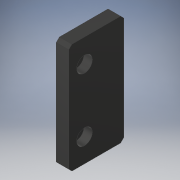
# Autodesk Inventor part: BT503_trajan20_21
Saved by Autodesk Inventor 2022.2 (Build 262287000, 287)
## iProperties
Company: HTBLA Kaindorf
RuleStatus: InUse
Created: 2022-08-19
Part Number: BT503_trajan20_21
Project: Zeichenmaschine_v2
Material: Kunststoff, undurchsichtig Schwarz
Description: Stifthalter_platte
Document SubType Name: Modeling
Designer: trajan20
Density: 0.952 g/cm^3
Appearance: Glatt - Schwarz
Mass: 17.4692 g
Surface Area: 70.5744 cm^2
Volume: 18.35 cm^3
AfterDocNew0: iProperties-Editor_aufrufen
Author: jan
Keywords: 2021
Autodesk Inventor part; units mm, degrees
ref_plane "YZ Plane" through (0, 0, 0) normal (1, 0, 0) x (0, 1, 0)
ref_plane "XZ Plane" through (0, 0, 0) normal (0, 1, 0) x (-1, 0, 0)
ref_plane "XY Plane" through (0, 0, 0) normal (0, 0, 1) x (1, 0, 0)
sketch "Skizze3" plane through (0, 0, 0) normal (0, 1, 0) x (-1, 0, 0)
  line L0 (0, 0) -> (0, -70)
  line L1 (0, -70) -> (35, -70)
  line L2 (35, -70) -> (35, 0)
  line L3 (35, 0) -> (0, 0)
  point P0 (30, -25)
  point P1 (30, -45)
  point P2 (35, -35)
  point P3 (10, -15)
  point P4 (10, -55)
  dimension "d4" = 35
  dimension "d5" = 70
  dimension "d6" = 5
  dimension "d7" = 5
  dimension "d8" = 10
  dimension "d9" = 10
  dimension "d10" = 15
  dimension "d11" = 15
  dimension "d12" = 10
  dimension "d13" = 10
  constraints: 8 end point, 3 perpendicular, 1 midpoint, 1 vertical
  measures "d4" distance between parallel lines of L2 L0
  measures "d5" distance between parallel lines of L3 L1
  measures "d6" distance from line of L2 point (30, -45)
  measures "d7" distance from line of L2 point (30, -25)
  measures "d8" vertical distance of point (35, -35) point (30, -25)
  measures "d9" vertical distance of point (35, -35) point (30, -45)
  measures "d10" distance from line of L1 point (10, -55)
  measures "d11" distance from line of L3 point (10, -15)
  measures "d12" distance from line of point (10, -15) L0
  measures "d13" distance from line of L0 point (10, -55)
extrude "Extrusion3" add sketch "Skizze3" along normal blind 8
hole "Bohrung1" at (-30, 0, -45) at (-30, 0, -25) direction (0, 1, 0) diameter 5 depth 6
sketch "Skizze4" plane through (0, 8, 0) normal (0, 1, 0) x (1, 0, 0)
  point P0 (0, 0)
  point P1 (-10, 15)
  point P2 (-10, 55)
  point P3 (-10, 15)
  point P4 (-10, 55)
  constraints: 2 coincident
hole "Bohrung2" at (-10, 8, -15) at (-10, 8, -55) direction (0, -1, 0) diameter 5 end through all counterbore diameter 10 counterbore depth 5.4
chamfer "Fase1" distance 2 angle 45 4 edges at (-35, 4, 0) (0, 4, 0) (0, 4, -70) (-35, 4, -70)
